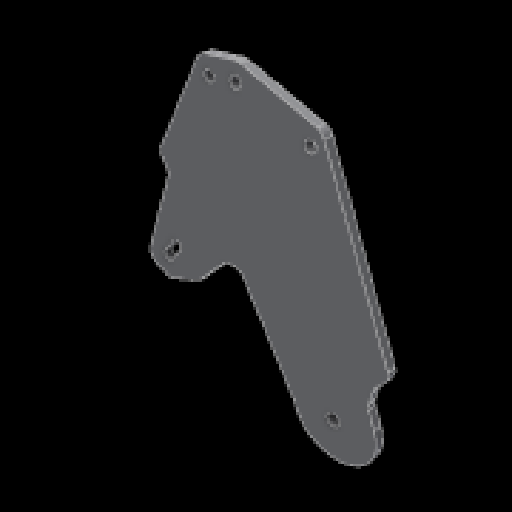
# Autodesk Inventor part: Knee
Saved by Autodesk Inventor 2025.2 (Build 292293000, 293)
## iProperties
Created: 2020-05-16
Part Number: Knee
Material: Generic
Document SubType Name: Sheet Metal
Designer: valer
Density: 1 g/cm^3
Sheet Metal Rule: Default
Appearance: Default
Author: valer
Autodesk Inventor part; units mm, degrees
ref_plane "YZ Plane" through (0, 0, 0) normal (1, 0, 0) x (0, 1, 0)
ref_plane "XZ Plane" through (0, 0, 0) normal (0, 1, 0) x (-1, 0, 0)
ref_plane "XY Plane" through (0, 0, 0) normal (0, 0, 1) x (1, 0, 0)
sketch "Base" plane through (0, 0, 0) normal (0, 0, 1) x (1, 0, 0)
  line L0 (0, 0) -> (-33.5334, -57.9479)
  line L1 (22.7363, 2.3748) -> (0, 0)
  line L2 (68.7163, -13.2577) -> (22.7363, 2.3748)
  line L3 (-33.5334, -57.9479) -> (-26.9158, -67.5067)
  line L4 (-26.9158, -67.5067) -> (-51.547, -128.5125)
  line L5 (-51.547, -128.5125) -> (-33.4114, -135.8348)
  line L6 (-26.9158, -67.5067) -> (12.6221, -101.6388) construction
  line L7 (12.6221, -101.6388) -> (22.7363, -101.0656)
  line L8 (12.6221, -101.6388) -> (-8.1441, -124.1457)
  line L9 (-33.4114, -135.8348) -> (-8.1441, -124.1457)
  line L10 (22.7363, 2.3748) -> (68.7163, -13.2577)
  line L11 (68.7163, -13.2577) -> (112.7039, -111.8391)
  line L12 (22.7363, 2.3748) -> (22.7363, -101.0656) construction
  line L13 (22.7363, -101.0656) -> (65.9464, -171.4033)
  line L14 (112.7039, -111.8391) -> (105.2475, -122.1197)
  line L15 (22.7363, -101.0656) -> (112.7039, -111.8391) construction
  line L16 (105.2475, -122.1197) -> (103.571, -134.8197)
  line L17 (103.571, -134.8197) -> (108.4402, -146.5492)
  line L18 (65.9464, -171.4033) -> (74.9694, -180.3406)
  line L19 (108.4402, -146.5492) -> (74.9694, -180.3406)
  circle A0 centre (85.3652, -157.1655) radius 25.4
  line L20 (-42.4792, -132.1736) -> (22.7363, -49.3454) construction
  line L21 (-33.0514, -120.1997) -> (-25.1949, -110.2215) construction
  line L22 (-35.546, -118.2356) -> (-27.6895, -108.2573)
  line L23 (-22.7004, -112.1856) -> (-30.5568, -122.1638)
  arc A1 (-35.546, -118.2356) -> (-30.5568, -122.1638) centre (-33.0514, -120.1997) ccw
  arc A2 (-22.7004, -112.1856) -> (-27.6895, -108.2573) centre (-25.1949, -110.2215) ccw
  circle A3 centre (85.3652, -157.1655) radius 4
  line L24 (0, -219.5535) -> (0, 39.3628)
  point P0 (-29.1232, -115.2106)
  point P1 (60.5618, -162.6381)
  dimension "d4" = 50.8
  dimension "d5" = 22.86
  dimension "d6" = 155.26
  dimension "d7" = 126.02
  dimension "d8" = 48.5647
  dimension "d9" = 66.9511
  dimension "d10" = 132.824
  dimension "d11" = 107.95
  dimension "d12" = 115.248
  dimension "d13" = 11.6259
  dimension "d14" = 65.7906
  dimension "d15" = 19.558
  dimension "d16" = 120
  dimension "d17" = 12.7
  dimension "d18" = 12.7
  dimension "d19" = 12.7
  dimension "d20" = 82.55
  dimension "d21" = 12.7
  dimension "d24" = 15.24
  dimension "d26" = 12.7
  dimension "d31" = 8
  dimension "d32" = 95.963
  dimension "d33" = 38.215
  dimension "d34" = 22.545
  dimension "d35" = 7.52
  dimension "d36" = 44.727
  dimension "d37" = 31.563
  dimension "d38" = 86.757
  dimension "d39" = 42.697
  dimension "d40" = 49.197
  dimension "d41" = 114.826
  dimension "d47" = 105.4209
  dimension "d48" = 62.051
  dimension "d75" = 3.175
  measures "d4" diameter of A0
  measures "d5" distance of L1.start L1.end
  measures "d6" angle of L2 L1
  measures "d7" angle of L0 L1
  measures "d8" distance of L2.start L1.start
  measures "d9" distance of L1.end L3.start
  measures "d10" angle of L2 L11
  measures "d11" distance of L2.start L11.end
  measures "d12" angle of L0 L3
  measures "d13" distance of L3.start L3.end
  measures "d14" distance of L3.end L4.end
  measures "d15" distance of L4.end L5.end
  measures "d16" angle of L14 L11
  measures "d17" distance of L11.end L16.start
  measures "d18" vertical distance of L16.start L16.end
  measures "d19" distance of L16.end L19.start
  measures "d20" distance of L7.end L13.end
  measures "d21" distance of L13.end L18.end
  measures "d24" distance of L20.start L21.start
  measures "d26" distance of L22.start L22.end
  measures "d31" diameter of A3
  measures "d32" angle of L24 L1
  measures "d33" angle of L24 L23
  measures "d34" angle of L17 L24
  measures "d35" angle of L16 L24
  measures "d36" angle of L19 L24
  measures "d37" angle of L13 L24
  measures "d38" angle of L7 L24
  measures "d39" angle of L8 L24
  measures "d40" angle of L6 L24
  measures "d41" angle of L9 L24
  measures "d47" distance of L20.start L20.end
  measures "d48" angle of L1 L4
  measures "d75" radius of A1
extrude "Plate1" add sketch "Base" along normal blind 5
fillet "OutsideFilletsFeature" radius 6.35 14 edges at (68.7163, -13.2577, 2.5) (22.7363, 2.3748, 2.5) (0, 0, 2.5) (-33.5334, -57.9479, 2.5) (-26.9158, -67.5067, 2.5) (-51.547, -128.5125, 2.5) (-33.4114, -135.8348, 2.5) (-8.1441, -124.1457, 2.5) (12.6221, -101.6388, 2.5) (22.7363, -101.0656, 2.5) (60.5618, -162.6381, 2.5) (103.571, -134.8197, 2.5) (105.2475, -122.1197, 2.5) (112.7039, -111.8391, 2.5)
sketch "MountHoles" plane through (0, 0, 5) normal (0, 0, 1) x (1, 0, 0)
  line L0 (-1.6199, -2.7989) -> (-30.9807, -53.5288) construction
  arc A0 (3.2163, 0.3359) -> (-1.6199, -2.7989) centre (3.876, -5.9797) ccw construction
  line L1 (21.3511, 2.2301) -> (3.2163, 0.3359) construction
  arc A1 (24.0549, 1.9264) -> (21.3511, 2.2301) centre (22.0108, -4.0856) ccw construction
  arc A2 (69.8461, -15.7897) -> (66.0912, -12.3652) centre (64.0472, -18.3772) ccw construction
  line L2 (24.0548, 1.9265) -> (66.0912, -12.3652) construction
  line L3 (66.0912, -12.3652) -> (24.0548, 1.9265) construction
  line L4 (-20.7142, -54.4632) -> (5.7075, -8.8047) construction
  line L5 (5.7075, -8.8047) -> (21.6681, -7.1377) construction
  line L6 (21.6681, -7.1377) -> (66.0912, -22.2408) construction
  line L7 (-31.5169, -54.4632) -> (-1.6198, -2.7992) construction
  line L8 (3.2166, 0.336) -> (21.3512, 2.2301) construction
  line L9 (24.0548, 1.9265) -> (66.0912, -12.3652) construction
  line L10 (-31.5169, -54.4632) -> (-20.7142, -54.4632) construction
  line L11 (66.0912, -22.2408) -> (66.0912, -12.3652) construction
  circle A3 centre (5.7075, -8.8047) radius 3
  circle A4 centre (21.6681, -7.1377) radius 3
  circle A5 centre (63.2509, -21.2751) radius 3
  point P0 (0, 0)
  dimension "d49" = 9.35
  dimension "d50" = 9.35
  dimension "d51" = 9.35
  dimension "d52" = 6
  dimension "d53" = 6
  dimension "d54" = 6
  dimension "d55" = 3
  constraints: 10 end point, 3 centre point, 3 parallel, 2 coincident, 1 horizontal, 1 perpendicular, 1 point on line
  measures "d49" distance between parallel lines of L4 L7
  measures "d50" distance between parallel lines of L1 L5
  measures "d51" distance between parallel lines of L2 L6
  measures "d52" diameter of A3
  measures "d53" diameter of A4
  measures "d54" diameter of A5
  measures "d55" distance of L6.end A5.centre
extrude "MountHolesFeature" cut sketch "MountHoles" against normal blind 5
equation "\"d50\" = d49"
equation "\"d51\" = d49"
equation "\"d56\" = Thickness"
equation "\"d42\" = Thickness"
equation "\"BendRadius\" = Thickness"
equation "\"BendReliefWidth\" = Thickness"
equation "\"BendReliefDepth\" = 0.5 * Thickness"
equation "\"TransitionRadius\" = BendRadius"
equation "\"JacobiRadiusSize\" = BendRadius"
equation "\"GapSize\" = Thickness"
equation "\"Thickness\" = 5"
body "Solid1"
